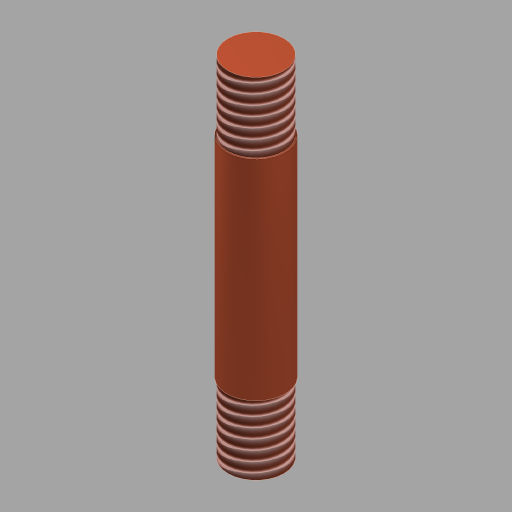
# Autodesk Inventor part: FrameSupport-Link
Saved by Autodesk Inventor 2024 (Build 280153020, 153B)
## iProperties
Created: 2023-08-18
Part Number: FrameSupport-Link
Material: Copper
Document SubType Name: Modeling
Designer: schanen
Density: 8.94 g/cm^3
Appearance: Copper - Satin
Author: schanen
Autodesk Inventor part; units mm, degrees
ref_plane "YZ Plane" through (0, 0, 0) normal (1, 0, 0) x (0, 1, 0)
ref_plane "XZ Plane" through (0, 0, 0) normal (0, 1, 0) x (-1, 0, 0)
ref_plane "XY Plane" through (0, 0, 0) normal (0, 0, 1) x (1, 0, 0)
sketch "Sketch1" plane through (0, 0, 0) normal (0, 0, 1) x (1, 0, 0)
  line L0 (0, 0) -> (-2, 0)
  line L1 (-2, 25) -> (0, 25)
  line L2 (0, 25) -> (0, 0)
  line L3 (-2, 25) -> (-2, 20)
  line L4 (-2, 20) -> (-2.1, 20)
  line L5 (-2.1, 20) -> (-2.1, 5)
  line L6 (-2.1, 5) -> (-2, 5)
  line L7 (-2, 5) -> (-2, 0)
  dimension "d0" = 2
  dimension "d7" = 2.1
  dimension "d12" = 5
  dimension "d13" = 5
  dimension "d14" = 25
  constraints: 16 end point, 4 perpendicular, 2 vertical, 1 horizontal, 1 parallel, 1 point on line
  measures "d0" distance of L1.start L1.end
  measures "d7" distance from line of L0.start L5
  measures "d12" distance of L6.end L0.end
  measures "d13" distance of L1.start L3.end
  measures "d14" distance of L1.end L0.start
revolve "Revolution1" add sketch "Sketch1" angle 360 about axis through (0, 25, 0) along (0, -1, 0)
thread "Thread2" size "M4x0.7" class "6g" standard "ANSI Metric M Profile" full length
body "Solid1"
